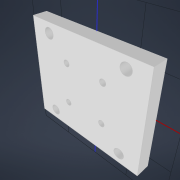
# Autodesk Inventor part: Master
Saved by Autodesk Inventor 2022 (Build 260153000, 153)
## iProperties
Created: 2021-06-27
Part Number: Master
Material: Generic
Document SubType Name: Modeling
Designer: user
Density: 1 g/cm^3
Appearance: Default
Author: user
Autodesk Inventor part; units mm, degrees
ref_plane "YZ Plane" through (0, 0, 0) normal (1, 0, 0) x (0, 1, 0)
ref_plane "XZ Plane" through (0, 0, 0) normal (0, 1, 0) x (-1, 0, 0)
ref_plane "XY Plane" through (0, 0, 0) normal (0, 0, 1) x (1, 0, 0)
sketch "Sketch2" plane through (0, 0, 0) normal (0, 1, 0) x (-1, 0, 0)
  line L0 (-10, 10) -> (10, 10) construction
  line L1 (10, 10) -> (10, -10) construction
  line L2 (10, -10) -> (-10, -10) construction
  line L3 (-10, -10) -> (-10, 10) construction
  line L4 (-10, 10) -> (10, -10) construction
  line L5 (10, 10) -> (-10, -10) construction
  line L6 (-20, 20) -> (20, 20) construction
  line L7 (20, 20) -> (20, -20) construction
  line L8 (20, -20) -> (-20, -20) construction
  line L9 (-20, -20) -> (-20, 20) construction
  line L10 (-20, 20) -> (20, -20) construction
  line L11 (20, 20) -> (-20, -20) construction
  line L12 (-30, 25) -> (30, 25)
  line L13 (30, 25) -> (30, -25)
  line L14 (30, -25) -> (-30, -25)
  line L15 (-30, -25) -> (-30, 25)
  line L16 (-30, 25) -> (30, -25) construction
  line L17 (30, 25) -> (-30, -25) construction
  circle A0 centre (-20, -20) radius 2.6
  circle A1 centre (20, -20) radius 2.6
  circle A2 centre (20, 20) radius 2.6
  circle A3 centre (-20, 20) radius 2.6
  circle A4 centre (-10, -10) radius 1.6
  circle A5 centre (10, -10) radius 1.6
  circle A6 centre (10, 10) radius 1.6
  circle A7 centre (-10, 10) radius 1.6
  point P0 (0, 0)
  dimension "d7" = 40
  dimension "d8" = 60
  dimension "d9" = 20
  dimension "d10" = 5.2
  dimension "d11" = 3.2
  dimension "d17" = 50
  constraints: 36 end point, 8 centre point, 8 coincident, 6 equal radius, 6 midpoint, 6 parallel, 5 perpendicular, 3 horizontal
  measures "d7" distance of L7.end L8.end
  measures "d8" distance of L13.end L14.end
  measures "d9" distance of L1.end L2.end
  measures "d10" diameter of A0
  measures "d11" diameter of A4
  measures "d17" distance of L12.end L13.end
extrude "Extrusion2" add sketch "Sketch2" along normal blind 7
sketch "Sketch3" plane through (-30, 0, 25) normal (0, 0, 1) x (1, 0, 0)
  circle A0 centre (30, 3.5) radius 1.6
  line L0 (0, 0) -> (60, 0) projected
  line L1 (60, 0) -> (60, 7) projected
  point P0 (30, 0)
  point P1 (30, 0)
  point P2 (60, 3.5)
  dimension "d14" = 3.2
  constraints: 2 midpoint, 1 centre point, 1 horizontal alignment, 1 vertical alignment
  measures "d14" diameter of A0
extrude "Extrusion3" [suppressed]
body "Solid2"
